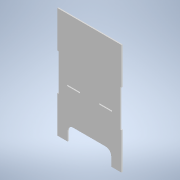
# Autodesk Inventor part: Pared_Lateral
Saved by Autodesk Inventor 2020.1 (Build 241239000, 239)
## iProperties
Created: 2019-12-08
Part Number: Pared_Lateral
Material: Generic
Document SubType Name: Modeling
Designer: Daniel
Density: 1 g/cm^3
Appearance: Default
Author: Daniel
Autodesk Inventor part; units mm, degrees
ref_plane "YZ Plane" through (0, 0, 0) normal (1, 0, 0) x (0, 1, 0)
ref_plane "XZ Plane" through (0, 0, 0) normal (0, 1, 0) x (-1, 0, 0)
ref_plane "XY Plane" through (0, 0, 0) normal (0, 0, 1) x (1, 0, 0)
sketch "Sketch1" plane through (0, 0, 0) normal (0, 0, 1) x (1, 0, 0)
  line L0 (-84, -131.5) -> (84, -131.5)
  line L1 (84, -131.5) -> (84, 168.5)
  line L2 (84, 168.5) -> (-84, 168.5)
  line L3 (-84, 168.5) -> (-84, -131.5)
  line L4 (-84, 1.5) -> (-84, -1.5) projected
  line L5 (84, -1.5) -> (84, 1.5) projected
  line L6 (61, -1.5) -> (84, -1.5) projected
  line L7 (26, -1.5) -> (61, -1.5) projected
  line L8 (61, 1.5) -> (61, -1.5) projected
  line L9 (26, 1.5) -> (61, 1.5) projected
  line L10 (26, 1.5) -> (26, -1.5) projected
  point P0 (0, 0)
  dimension "d0" = 300
  dimension "d1" = 170
  constraints: 8 end point, 2 collinear, 2 parallel, 1 horizontal, 1 perpendicular
  measures "d0" distance of L0.end L1.end
  measures "d1" distance between parallel lines of L2 L6
extrude "Extrusion1" add sketch "Sketch1" along normal blind 3
sketch "Sketch2" plane through (0, 0, 0) normal (0, 0, -1) x (-1, 0, 0)
  line L0 (84, 1.5) -> (84, -1.5)
  line L1 (84, -1.5) -> (61, -1.5)
  line L2 (61, 1.5) -> (61, -1.5)
  line L3 (26, 1.5) -> (61, 1.5)
  line L4 (26, -1.5) -> (26, 1.5)
  line L5 (26, -1.5) -> (-26, -1.5)
  line L6 (-26, 1.5) -> (-26, -1.5)
  line L7 (-61, 1.5) -> (-26, 1.5)
  line L8 (-61, -1.5) -> (-61, 1.5)
  line L9 (-61, -1.5) -> (-84, -1.5)
  line L10 (-84, -1.5) -> (-84, 1.5)
  line L11 (-84, 1.5) -> (-61, 1.5)
  line L12 (61, 1.5) -> (84, 1.5)
  line L13 (61, -1.5) -> (26, -1.5)
  line L14 (-26, 1.5) -> (26, 1.5)
  line L15 (-26, -1.5) -> (-61, -1.5)
  point P0 (0, 0)
  constraints: 32 end point, 10 horizontal, 6 vertical, 12 other
extrude "Extrusion2" cut sketch "Sketch2" against normal blind 10 contours L2 L13 L4 L3
sketch "Sketch3" plane through (0, 0, 3) normal (0, 0, 1) x (1, 0, 0)
  line L0 (84, -131.5) -> (84, 168.5) projected
  line L1 (84, -131.5) -> (87, -131.5)
  line L2 (87, -131.5) -> (87, -31.5)
  line L3 (87, -31.5) -> (84, -31.5)
  line L4 (84, -31.5) -> (84, -131.5)
  line L5 (-61, -1.5) -> (-26, -1.5) projected
  line L6 (-26, -1.5) -> (-26, 1.5) projected
  line L7 (-26, 1.5) -> (-61, 1.5) projected
  line L8 (-61, 1.5) -> (-61, -1.5) projected
  line L9 (26, 1.5) -> (26, -1.5) projected
  line L10 (26, -1.5) -> (61, -1.5) projected
  line L11 (61, -1.5) -> (61, 1.5) projected
  line L12 (61, 1.5) -> (26, 1.5) projected
  line L13 (-84, 168.5) -> (84, 168.5) projected
  line L14 (84, 168.5) -> (84, -131.5) projected
  line L15 (84, -131.5) -> (-84, -131.5) projected
  line L16 (-84, -131.5) -> (-84, 168.5) projected
  line L17 (87, 168.5) -> (84, 168.5)
  line L18 (84, 68.5) -> (87, 68.5)
  line L19 (87, 68.5) -> (87, 168.5)
  line L20 (84, 168.5) -> (84, 68.5)
  line L21 (-84, -31.5) -> (-87, -31.5)
  line L22 (-87, -131.5) -> (-84, -131.5)
  line L23 (-84, -131.5) -> (-84, -31.5)
  line L24 (-87, -31.5) -> (-87, -131.5)
  line L25 (-84, 168.5) -> (-87, 168.5)
  line L26 (-87, 68.5) -> (-84, 68.5)
  line L27 (-84, 68.5) -> (-84, 168.5)
  line L28 (-87, 168.5) -> (-87, 68.5)
  point P0 (0, 0)
  dimension "d6" = 100
  dimension "d7" = 3
  dimension "d10" = 200
  dimension "d13" = 171
  constraints: 32 end point, 2 horizontal, 2 parallel, 1 perpendicular, 1 vertical, 24 other
  measures "d6" distance of L1.end L2.end
  measures "d7" distance of L0.start L1.end
  measures "d10" distance of L3.end L17.end
  measures "d13" distance of L3.end L21.end
extrude "Extrusion3" add sketch "Sketch3" against normal up to surface (3 mm away) contours L0 L3 L2 L1 | L22 L24 L21 L16 | L0 L17 L19 L18 | L26 L28 L25 L16
sketch "Sketch4" plane through (0, 0, 3) normal (0, 0, 1) x (1, 0, 0)
  line L0 (-59, -131.5) -> (59, -131.5)
  line L1 (59, -131.5) -> (59, -91.5)
  line L2 (59, -91.5) -> (-59, -91.5)
  line L3 (-59, -91.5) -> (-59, -131.5)
  line L4 (-87, -131.5) -> (87, -131.5) projected
  line L5 (87, -131.5) -> (87, -31.5) projected
  line L6 (-87, -31.5) -> (-87, -131.5) projected
  point P0 (0, 0)
  dimension "d18" = 28
  dimension "d19" = 28
  dimension "d20" = 40
  constraints: 8 end point, 2 parallel, 1 collinear, 1 horizontal, 1 perpendicular
  measures "d18" distance between parallel lines of L5 L1
  measures "d19" distance between parallel lines of L6 L3
  measures "d20" distance of L0.end L1.end
extrude "Extrusion4" cut sketch "Sketch4" against normal blind 10
fillet "Fillet1" radius 15 2 edges at (59, -91.5, 1.5) (-59, -91.5, 1.5)
body "Solid1"
